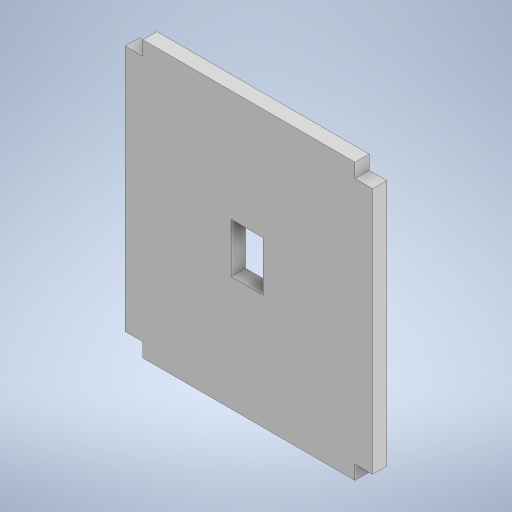
# Autodesk Inventor part: Knoptsnstuk_Final
Saved by Autodesk Inventor 2023.4 (Build 274418000, 418)
## iProperties
Created: 2024-08-06
Part Number: Knoptsnstuk_Final
Material: Generic
Document SubType Name: Modeling
Designer: cthey
Density: 1 g/cm^3
Appearance: Default
Author: cthey
Autodesk Inventor part; units mm, degrees
ref_plane "YZ Plane" through (0, 0, 0) normal (1, 0, 0) x (0, 1, 0)
ref_plane "XZ Plane" through (0, 0, 0) normal (0, 1, 0) x (-1, 0, 0)
ref_plane "XY Plane" through (0, 0, 0) normal (0, 0, 1) x (1, 0, 0)
sketch "Sketch1" plane through (0, 0, 0) normal (0, 0, 1) x (1, 0, 0)
  line L0 (0, 0) -> (70, 0)
  line L1 (70, 0) -> (70, 70)
  line L2 (70, 70) -> (0, 70)
  line L3 (0, 70) -> (0, 0)
  line L4 (5, 74) -> (65, 74)
  line L5 (65, 74) -> (65, -4)
  line L6 (65, -4) -> (5, -4)
  line L7 (5, -4) -> (5, 74)
  line L8 (30, 42.5) -> (39, 42.5)
  line L9 (39, 42.5) -> (39, 28.5)
  line L10 (39, 28.5) -> (30, 28.5)
  line L11 (30, 28.5) -> (30, 42.5)
  point P0 (5, 0)
  point P1 (65, 0)
  point P2 (65, 70)
  point P3 (5, 70)
  dimension "d0" = 70
  dimension "d1" = 70
  dimension "d2" = 4
  dimension "d3" = 5
  dimension "d4" = 5
  dimension "d5" = 4
  dimension "d6" = 14
  dimension "d7" = 9
  dimension "d8" = 26
  dimension "d9" = 28.5
  constraints: 24 end point, 6 parallel, 3 horizontal, 3 perpendicular
  measures "d0" distance of L1.end L2.end
  measures "d1" distance of L0.end L1.end
  measures "d2" distance between parallel lines of L2 L4
  measures "d3" distance between parallel lines of L1 L5
  measures "d4" distance between parallel lines of L3 L7
  measures "d5" distance between parallel lines of L0 L6
  measures "d6" distance of L8.end L9.end
  measures "d7" distance of L8.start L8.end
  measures "d8" distance between parallel lines of L5 L9
  measures "d9" distance between parallel lines of L0 L10
extrude "Extrusion1" add sketch "Sketch1" along normal blind 4
body "Solid1"
